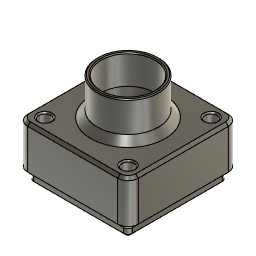
Gridfinity Engineer SS-02 stand v5 (Autodesk Fusion 360 design; units mm, degrees)
Autodesk Fusion 360 part; units mm, degrees
sketch "Sketch1" plane through (0, 0, 0) normal (0, 0, 1) x (1, 0, 0) in component "Gridfinity bin 1x1x0"
  line L0 (0, 0) -> (41.8, 0)
  line L1 (41.8, 0) -> (41.8, 41.8)
  line L2 (41.8, 41.8) -> (0, 41.8)
  line L3 (0, 41.8) -> (0, 0)
  dimension "d1" = 41.8
  dimension "d2" = 41.8
  constraint horizontal L0
  constraint vertical L1
  constraint horizontal L2
  constraint vertical L3
  constraint coincident L0.start L3
  constraint coincident L3.end L0
  measures "d1" horizontal distance of L0.start L0.end
  measures "d2" vertical distance of L0.end L1.end
extrude "Extrude1" add sketch "Sketch1" against normal blind 2.3 makes body 1 in component "Gridfinity bin 1x1x0"
fillet "Fillet1" radius 3.9 4 edges at (0, 0, -1.15) (41.8, 0, -1.15) (41.8, 41.8, -1.15) (0, 41.8, -1.15) on bodies 1 in component "Gridfinity bin 1x1x0"
chamfer "Chamfer1" distance 2.3 angle 45 8 edges at (1.1423, 40.6577, -2.3) (0, 20.9, -2.3) (1.1423, 1.1423, -2.3) (20.9, 0, -2.3) (40.6577, 1.1423, -2.3) (41.8, 20.9, -2.3) (40.6577, 40.6577, -2.3) (20.9, 41.8, -2.3) on bodies 1 in component "Gridfinity bin 1x1x0"
extrude "Extrude2" add 1 faces at (26.5667, 14.6998, -2.3) along direction (0, 0, -1) blind 2.7 on bodies 1 bodies 1 in component "Gridfinity bin 1x1x0"
chamfer "Chamfer2" distance 0.8 angle 45 8 edges at (2.7686, 39.0314, -5) (20.9, 39.5, -5) (39.0314, 39.0314, -5) (39.5, 20.9, -5) (39.0314, 2.7686, -5) (20.9, 2.3, -5) (2.7686, 2.7686, -5) (2.3, 20.9, -5) on bodies 1 in component "Gridfinity bin 1x1x0"
hole "Hole1" at (8, 8, 0) direction (0, 0, -1) diameter 3 end through all bodies 1 in component "Gridfinity bin 1x1x0"
sketch "Sketch2" plane through (0, 0, -5) normal (0, 0, -1) x (-1, 0, 0) in component "Gridfinity bin 1x1x0"
  circle A0 centre (-8, 8) radius 1.5 construction
  arc A1 (-3.1, 37.9) -> (-3.9, 38.7) centre (-3.9, 37.9) ccw construction
  line L0 (-3.9, 38.7) -> (-37.9, 38.7) construction
  arc A2 (-37.9, 38.7) -> (-38.7, 37.9) centre (-37.9, 37.9) ccw construction
  line L1 (-38.7, 37.9) -> (-38.7, 3.9) construction
  arc A3 (-38.7, 3.9) -> (-37.9, 3.1) centre (-37.9, 3.9) ccw construction
  line L2 (-37.9, 3.1) -> (-3.9, 3.1) construction
  arc A4 (-3.9, 3.1) -> (-3.1, 3.9) centre (-3.9, 3.9) ccw construction
  line L3 (-3.1, 3.9) -> (-3.1, 37.9) construction
  circle A5 centre (-8, 8) radius 3.25
  dimension "d16" = 6.5
  dimension "d17" = 8
  dimension "d18" = 8
  measures "d16" diameter of A5
  measures "d17" horizontal distance of origin A0.centre
  measures "d18" vertical distance of origin A0.centre
extrude "Extrude3" cut sketch "Sketch2" against normal blind 2.4 bodies 1 in component "Gridfinity bin 1x1x0"
sketch "Sketch3" plane through (0, 0, -2.6) normal (0, 0, -1) x (-1, 0, 0) in component "Gridfinity bin 1x1x0"
  circle A0 centre (-8, 8) radius 1.5 construction
  circle A1 centre (-8, 8) radius 3.25 construction
  line L0 (-5.1169, 6.5) -> (-10.8831, 6.5)
  line L1 (-5.1169, 9.5) -> (-10.8831, 9.5)
  arc A2 (-5.1169, 6.5) -> (-5.1169, 9.5) centre (-8, 8) ccw
  arc A3 (-10.8831, 9.5) -> (-10.8831, 6.5) centre (-8, 8) ccw
  constraint coincident L1.start A2.end
  constraint coincident L0.end A3.end
  constraint concentric A0 A2
  constraint concentric A0 A3
  constraint tangent A0 L0
  constraint tangent A0 L1
  constraint coincident A1 L1.start
  constraint coincident A1 L1.end
  constraint horizontal L0
  constraint horizontal L1
extrude "Extrude4" cut sketch "Sketch3" against normal blind 0.3 bodies 1 in component "Gridfinity bin 1x1x0"
pattern_linear "R-Pattern1" count 2 spacing 26 along (1, 0, 0) count 2 spacing 26 along (0, 1, 0) of "Hole1", "Extrude3", "Extrude4" in component "Gridfinity bin 1x1x0"
pattern_linear "R-Pattern2" count 1 spacing 42 along (1, 0, 0) of bodies 1 merged in component "Gridfinity bin 1x1x0"
sketch "Sketch4" plane through (0, 0, 0) normal (0, 0, 1) x (1, 0, 0) in component "Gridfinity bin 1x1x0"
  line L0 (0, 0) -> (41.8, 0)
  line L1 (41.8, 0) -> (41.8, 41.8)
  line L2 (41.8, 41.8) -> (0, 41.8)
  line L3 (0, 41.8) -> (0, 0)
  dimension "d31" = 41.8
  dimension "d32" = 41.8
  constraint horizontal L0
  constraint vertical L1
  constraint horizontal L2
  constraint vertical L3
  constraint coincident L0.start L3
  constraint coincident L3.end L0
  measures "d31" horizontal distance of L0.start L0.end
  measures "d32" vertical distance of L0.end L1.end
extrude "Extrude5" add sketch "Sketch4" along normal blind 16 separate body makes body 2 in component "Gridfinity bin 1x1x0"
fillet "Fillet2" radius 3.9 8 edges at (41.8, 41.8, 8) (41.8, 0, 8) (41.8, 0, 8) (0, 0, 8) (0, 0, 8) (0, 41.8, 8) (0, 41.8, 8) (41.8, 41.8, 8) on bodies 2 in component "Gridfinity bin 1x1x0"
combine "Combine1" operation add target body 2 tool bodies 1 in component "Gridfinity bin 1x1x0"
chamfer "Chamfer3" distance 1 angle 45 8 edges at (41.8, 20.9, 16) (40.6577, 40.6577, 16) (20.9, 41.8, 16) (1.1423, 40.6577, 16) (0, 20.9, 16) (1.1423, 1.1423, 16) (20.9, 0, 16) (40.6577, 1.1423, 16) on bodies 2 in component "Gridfinity bin 1x1x0"
sketch "Sketch5" plane through (0, 0, 16) normal (0, 0, 1) x (-1, 0, 0) in component "Gridfinity bin 1x1x0"
  line L0 (-40.8, -3.9) -> (-40.8, -37.9)
  arc A0 (-40.8, -37.9) -> (-37.9, -40.8) centre (-37.9, -37.9) ccw
  line L1 (-37.9, -40.8) -> (-3.9, -40.8)
  arc A1 (-3.9, -40.8) -> (-1, -37.9) centre (-3.9, -37.9) ccw
  line L2 (-1, -37.9) -> (-1, -3.9)
  arc A2 (-1, -3.9) -> (-3.9, -1) centre (-3.9, -3.9) ccw
  line L3 (-3.9, -1) -> (-37.9, -1)
  arc A3 (-37.9, -1) -> (-40.8, -3.9) centre (-37.9, -3.9) ccw
  circle A4 centre (-20.9, -20.9) radius 11.5
  circle A5 centre (-20.9, -20.9) radius 6
  dimension "d38" = 23
  dimension "d41" = 12
  constraint concentric A4 A5
  measures "d38" diameter of A4
  measures "d41" diameter of A5
extrude "Extrude7" cut sketch "Sketch5" against normal blind 20 contours A5 bodies 2 in component "Gridfinity bin 1x1x0"
extrude "Extrude6" add sketch "Sketch5" along normal blind 14 contours A4 | A5 bodies 2 in component "Gridfinity bin 1x1x0"
hole "Hole2" at (20.9, 20.9, 30) direction (0, 0, -1) diameter 20.2 depth 11 tip angle 72 bodies 2 in component "Gridfinity bin 1x1x0"
chamfer "Chamfer4" distance 1 angle 45 1 edges at (26.494, 18.7303, -4) on bodies 2 in component "Gridfinity bin 1x1x0"
chamfer "Chamfer5" distance 2.5 angle 45 1 edges at (31.6218, 16.7414, 16) on bodies 2 in component "Gridfinity bin 1x1x0"
sketch "Sketch6" plane through (0, 0, 16) normal (0, 0, 1) x (-1, 0, 0) in component "Gridfinity bin 1x1x0"
  line L0 (-40.8, -3.9) -> (-40.8, -37.9)
  arc A0 (-40.8, -37.9) -> (-37.9, -40.8) centre (-37.9, -37.9) ccw
  line L1 (-37.9, -40.8) -> (-3.9, -40.8)
  arc A1 (-3.9, -40.8) -> (-1, -37.9) centre (-3.9, -37.9) ccw
  line L2 (-1, -37.9) -> (-1, -3.9)
  arc A2 (-1, -3.9) -> (-3.9, -1) centre (-3.9, -3.9) ccw
  line L3 (-3.9, -1) -> (-37.9, -1)
  arc A3 (-37.9, -1) -> (-40.8, -3.9) centre (-37.9, -3.9) ccw
  circle A4 centre (-20.9, -20.9) radius 14
  line L4 (-40.8, -1) -> (-36.6, -1) construction
  line L5 (-36.6, -1) -> (-36.6, -5.2) construction
  line L6 (-36.6, -5.2) -> (-40.8, -5.2) construction
  line L7 (-40.8, -5.2) -> (-40.8, -1) construction
  line L8 (-1, -1) -> (-5.2, -1) construction
  line L9 (-5.2, -1) -> (-5.2, -5.2) construction
  line L10 (-5.2, -5.2) -> (-1, -5.2) construction
  line L11 (-1, -5.2) -> (-1, -1) construction
  line L12 (-1, -40.8) -> (-5.2, -40.8) construction
  line L13 (-5.2, -40.8) -> (-5.2, -36.6) construction
  line L14 (-5.2, -36.6) -> (-1, -36.6) construction
  line L15 (-1, -36.6) -> (-1, -40.8) construction
  point P0 (-36.6, -5.2)
  point P1 (-51.2616, -10.2466)
  point P2 (-5.2, -5.2)
  point P3 (-36.6, -36.6)
  point P4 (-5.2, -36.6)
  dimension "d49" = 4.2
  dimension "d50" = 4.2
  dimension "d53" = 31.4
  dimension "d54" = -31.4
  dimension "d55" = 4.2
  dimension "d56" = 4.2
  dimension "d57" = 4.2
  dimension "d58" = 4.2
  constraint horizontal L4
  constraint vertical L5
  constraint horizontal L6
  constraint vertical L7
  constraint coincident P0 L5.end
  constraint horizontal L8
  constraint vertical L9
  constraint horizontal L10
  constraint vertical L11
  constraint horizontal L12
  constraint vertical L13
  constraint horizontal L14
  constraint vertical L15
  measures "d49" distance of L4.start L4.end
  measures "d50" distance of L4.start L6.end
  measures "d55" distance of L8.start L8.end
  measures "d56" distance of L8.start L10.end
  measures "d57" distance of L12.start L12.end
  measures "d58" distance of L12.start L14.end
hole "Hole3" at (5.2, 5.2, 16) at (36.6, 5.2, 16) at (36.6, 36.6, 16) at (5.2, 36.6, 16) direction (0, 0, -1) diameter 4.5 depth 12 tip angle 118 bodies 2 in component "Gridfinity bin 1x1x0"
chamfer "Chamfer6" distance 0.5 angle 45 4 edges at (3.1023, 37.4136, 16) (34.5023, 37.4136, 16) (34.5023, 6.0136, 16) (3.1023, 6.0136, 16) on bodies 2 in component "Gridfinity bin 1x1x0"
chamfer "Chamfer7" distance 0.35 angle 45 2 edges at (31.6218, 25.0586, 30) (11.4835, 24.5523, 30) on bodies 2 in component "Gridfinity bin 1x1x0"
cylinder "CylinderPrimitive1" add diameter 19.9 height 51 placed x (1, 0, 0) y (0, 1, 0) z (0, 0, 1) at (65, 21, 0) separate body makes body 3
chamfer "Chamfer1'" distance 5.5 angle 54 1 edges at (55.7233, 24.5981, 0) measured on face at (63.0132, 22.4333, 0) on bodies 3
cylinder "CylinderPrimitive2" add diameter 6.9 height 15 placed x (0, 1, 0) y (1, 0, 0) z (0, 0, -1) at (65, 21, 0) bodies 3
move_body "Move1" bodies 3 to x (1, 0, 0) y (0, 1, 0) z (0, 0, 1) at (-44.1, -0.1, 13.3568)
move_body "Move2" bodies 3 to x (1, 0, 0) y (0, 1, 0) z (0, 0, 1) at (0, 0, -1.95)
component "Gridfinity bin 1x1x0" placed x (1, 0, 0) y (0, 1, 0) z (0, 0, 1) at (0, 0, 0)
hidden bodies 3
equation "d3 = -( 2.30 mm )"
equation "d19 = -( 2.40 mm )"
equation "d21 = -( 0.30 mm )"
named bodies: "base", "Gridfinity bin 1x1x0"
